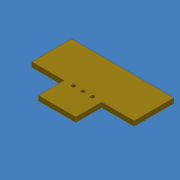
# Autodesk Inventor part: Sharp GP2Y0 Sensor PCB
Saved by Autodesk Inventor 2012 (Build 160160000, 160)
## iProperties
Category: FIRST
Manager: Ed Sparks
Company: FirstCadLibrary
Shininess: 64.0
Length Units: 11269
Angle Units: 11279
Time Units: 11290
Mass Units: 11283
Length Display Precision: 3
Angle Display Precision: 2
Compacted: True
Part Number: Sharp GP2Y0 Sensor PCB
Document SubType Name: Modeling
Created: 2007-12-20
Material: Phenolic
Designer: Ed Sparks
Catalog Web Link: www.firstcadlibrary.com
Engineer: Ed Sparks
Density: 1.38 g/cm^3
Mass: 0.660898 g
Surface Area: 8.6747 cm^2
Volume: 0.478912 cm^3
Density: 0.0
Volumn: 0.0
Area: 0.0
PropertySet Name: Model Information
Control State: 0
Master: False
Checked Out: False
Author: Ed Sparks
Keywords: FIRST
Autodesk Inventor part; units mm, degrees
ref_plane "YZ Plane" through (0, 0, 0) normal (1, 0, 0) x (0, 1, 0)
ref_plane "XZ Plane" through (0, 0, 0) normal (0, 1, 0) x (-1, 0, 0)
ref_plane "XY Plane" through (0, 0, 0) normal (0, 0, 1) x (1, 0, 0)
sketch "Sketch1" plane through (0, 0, 0) normal (0, 0, 1) x (1, 0, 0)
  line L0 (-13.875, 5.4) -> (13.875, 5.4)
  line L1 (13.875, 5.4) -> (13.875, -5.4)
  line L2 (-13.875, -5.4) -> (-13.875, 5.4)
  line L3 (0, 0) -> (0, -5.4) construction
  line L4 (0, 0) -> (13.875, 0) construction
  line L5 (0, 0) -> (-13.875, 0) construction
  line L6 (-5.075, -5.4) -> (-5.075, -12.4)
  line L7 (-5.075, -12.4) -> (5.075, -12.4)
  line L8 (5.075, -12.4) -> (5.075, -5.4)
  line L9 (13.875, -5.4) -> (5.075, -5.4)
  line L10 (-5.075, -5.4) -> (-13.875, -5.4)
  dimension "d0" = 27.75
  dimension "d1" = 10.8
  dimension "d2" = 10.15
  dimension "d3" = 7
  constraints: 22 end point, 3 parallel, 2 collinear, 2 horizontal, 2 midpoint, 2 vertical, 1 perpendicular, 3 other
  measures "d0" distance of L0.start L0.end
  measures "d1" distance of L0.end L1.end
  measures "d2" distance of L6.end L7.end
  measures "d3" distance between parallel lines of L7 L9
extrude "Extrusion1" add sketch "Sketch1" along normal mid plane 1.3
sketch "Sketch2" plane through (0, 0, 0.65) normal (0, 0, 1) x (1, 0, 0)
  line L0 (-13.875, 5.4) -> (13.875, 5.4) projected
  line L1 (5.075, -12.4) -> (-5.075, -12.4) projected
  line L2 (-5.075, -5.4) -> (5.075, -5.4) construction
  line L3 (0, -12.4) -> (0, 5.4) construction
  point P0 (-2.54, -5.4)
  point P1 (0, -5.4)
  point P2 (2.54, -5.4)
  dimension "d6" = 2.54
  dimension "d7" = 2.54
  constraints: 4 end point, 3 midpoint, 3 point on line, 1 horizontal
  measures "d6" distance of point (2.54, -5.4) point (0, -5.4)
  measures "d7" distance from line of L3 point (-2.54, -5.4)
hole "Hole1" at (-2.54, -5.4, 0.65) at (0, -5.4, 0.65) at (2.54, -5.4, 0.65) direction (0, 0, -1) diameter 1 end through all
body "Solid1"
